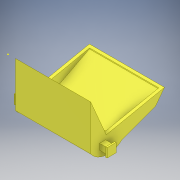
# Autodesk Inventor part: hoe me
Saved by Autodesk Inventor 2018 (Build 220112000, 112)
## iProperties
Created: 2018-01-20
Part Number: hoe me
Material: Generic
Document SubType Name: Modeling
Designer: omara
Density: 1 g/cm^3
Appearance: Smooth - Yellow
Author: omara
Autodesk Inventor part; units mm, degrees
ref_plane "YZ Plane" through (0, 0, 0) normal (1, 0, 0) x (0, 1, 0)
ref_plane "XZ Plane" through (0, 0, 0) normal (0, 1, 0) x (-1, 0, 0)
sketch "Sketch1" plane through (0, 0, 0) normal (1, 0, 0) x (0, 1, 0)
  line L0 (0, 0) -> (0, -300)
  line L1 (0, 0) -> (103.9616, -241.9966)
  line L2 (431.1742, -241.9966) -> (207.8735, -323.7914)
  arc A0 (0, -300) -> (207.8735, -323.7914) centre (114.5573, -219.1004) ccw
  line L3 (103.9616, -241.9966) -> (492.1494, -162.4552)
  line L4 (492.1494, -162.4552) -> (431.1742, -241.9966)
  dimension "d5" = 300
  constraints: 10 end point, 2 point on circle, 1 centre point, 1 vertical
  measures "d5" distance of L0.start L0.end
extrude "Extrusion1" add sketch "Sketch1" against normal blind 500
ref_plane "Work Plane1" through (-20, 0, 0) normal (1, 0, 0) x (0, 0, -1)
sketch "Sketch2" plane through (-20, 0, 0) normal (1, 0, 0) x (0, 0, -1)
  line L0 (292.8468, 11.7995) -> (-65.8674, 11.7995)
  line L1 (170.4104, 471.7728) -> (314.1993, 195.7664)
  arc A0 (290.3714, 11.7995) -> (314.1993, 195.7664) centre (219.1004, 114.5573) ccw
  arc A1 (300, 0) -> (323.7914, 207.8735) centre (219.1004, 114.5573) ccw projected
  line L2 (-61.2921, 11.7995) -> (-54.1186, 588.7001)
  line L3 (-54.1186, 588.7001) -> (170.4104, 471.7728)
  point P0 (0, 0)
  dimension "d9" = 250.1097
  constraints: 8 end point, 2 point on circle, 2 point on line, 1 centre point, 1 concentric, 1 horizontal
  measures "d9" diameter of A0
extrude "Extrusion2" cut sketch "Sketch2" against normal blind 460
sketch "Sketch3" plane through (0, 0, 0) normal (1, 0, 0) x (0, 0, -1)
  line L0 (269.1004, 100) -> (309.1004, 100)
  line L1 (309.1004, 100) -> (309.1004, 60)
  line L2 (309.1004, 60) -> (269.1004, 60)
  line L3 (269.1004, 60) -> (269.1004, 100)
  line L4 (0, 0) -> (300, 0) projected
  arc A0 (300, 0) -> (323.7914, 207.8735) centre (219.1004, 114.5573) ccw projected
  dimension "d12" = 40
  dimension "d13" = 40
  dimension "d14" = 60
  dimension "d15" = 90
  constraints: 8 end point, 2 parallel, 1 horizontal, 1 perpendicular
  measures "d12" distance of L1.end L2.end
  measures "d13" distance between parallel lines of L2 L0
  measures "d14" distance between parallel lines of L4 L2
  measures "d15" distance from line of A0.centre L1
extrude "Extrusion3" add sketch "Sketch3" along normal blind 50
sketch "Sketch4" plane through (50, 0, 0) normal (1, 0, 0) x (0, 0, -1)
  line L0 (309.1004, 100) -> (269.1004, 100) projected
  line L1 (269.1004, 100) -> (269.1004, 60) projected
  line L2 (269.1004, 60) -> (309.1004, 60) projected
  line L3 (309.1004, 60) -> (309.1004, 100) projected
  line L4 (259.1004, 110) -> (319.1004, 110)
  line L5 (319.1004, 110) -> (319.1004, 50)
  line L6 (319.1004, 50) -> (259.1004, 50)
  line L7 (259.1004, 50) -> (259.1004, 110)
  point P0 (0, 0)
  dimension "d18" = 60
  dimension "d19" = 60
  dimension "d20" = 10
  dimension "d21" = 10
  constraints: 8 end point, 2 parallel, 1 horizontal, 1 perpendicular
  measures "d18" distance between parallel lines of L6 L4
  measures "d19" distance between parallel lines of L5 L7
  measures "d20" distance between parallel lines of L0 L4
  measures "d21" distance between parallel lines of L5 L3
extrude "Extrusion4" add sketch "Sketch4" along normal blind 10 contours L3 L2 L1 L0 | L4 L5 L6 L7
sketch "Sketch5" plane through (-500, 0, 0) normal (-1, 0, 0) x (0, 0, 1)
  line L0 (-309.1004, 100) -> (-269.1004, 100)
  line L1 (-269.1004, 100) -> (-269.1004, 60)
  line L2 (-269.1004, 60) -> (-309.1004, 60)
  line L3 (-309.1004, 60) -> (-309.1004, 100)
  arc A0 (-323.7914, 207.8735) -> (-300, 0) centre (-219.1004, 114.5573) ccw projected
  line L4 (-300, 0) -> (0, 0) projected
  dimension "d24" = 40
  dimension "d25" = 40
  dimension "d26" = 90
  dimension "d27" = 60
  constraints: 8 end point, 2 parallel, 1 horizontal, 1 perpendicular
  measures "d24" distance of L1.end L2.end
  measures "d25" distance of L0.end L1.end
  measures "d26" distance from line of A0.centre L3
  measures "d27" distance between parallel lines of L4 L2
extrude "Extrusion5" add sketch "Sketch5" along normal blind 50
sketch "Sketch6" plane through (-550, 0, 0) normal (-1, 0, 0) x (0, 0, 1)
  point P0 (0, 0)
sketch "Sketch7" plane through (-550, 0, 0) normal (-1, 0, 0) x (0, 0, 1)
  point P0 (0, 0)
sketch "Sketch8" plane through (-550, 0, 0) normal (-1, 0, 0) x (0, 0, 1)
  line L0 (-269.1004, 100) -> (-309.1004, 100) projected
  line L1 (-309.1004, 100) -> (-309.1004, 60) projected
  line L2 (-309.1004, 60) -> (-269.1004, 60) projected
  line L3 (-269.1004, 60) -> (-269.1004, 100) projected
  line L4 (-319.1004, 110) -> (-259.1004, 110)
  line L5 (-259.1004, 110) -> (-259.1004, 50)
  line L6 (-259.1004, 50) -> (-319.1004, 50)
  line L7 (-319.1004, 50) -> (-319.1004, 110)
  point P0 (0, 0)
  dimension "d30" = 60
  dimension "d31" = 60
  dimension "d33" = 10
  dimension "d34" = 10
  constraints: 8 end point, 2 parallel, 1 horizontal, 1 perpendicular
  measures "d30" distance of L5.end L6.end
  measures "d31" distance of L4.end L5.end
  measures "d33" distance between parallel lines of L7 L1
  measures "d34" distance between parallel lines of L0 L4
extrude "Extrusion6" add sketch "Sketch8" along normal blind 10 contours L3 L2 L1 L0 | L4 L5 L6 L7
body "Solid1"
